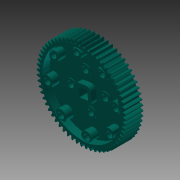
# Autodesk Inventor part: 276-2250
Saved by Autodesk Inventor 2013 (Build 170138000, 138)
## iProperties
Category: Motion
Company: Autodesk Inc.
Created: 2012-02-19
Part Number: 276-2250
Document SubType Name: Modeling
Designer: Autodesk Inc.
Density: 1.42 g/cm^3
Material: Acetal Resin, White
Catalog Web Link: http://www.vexrobotics.com/276-2250.html
Vendor: VEX
Mass: 21.4122 g
Surface Area: 169.555 cm^2
Volume: 15.079 cm^3
Author: Autodesk Inc.
Autodesk Inventor part; units mm, degrees
sketch "Sketch1" plane through (0, 0, 0) normal (0, 0, 1) x (1, 0, 0)
  arc A0 (28.1475, -11.53) -> (28.6057, -10.3412) centre (0, 0) ccw
  arc A1 (28.6057, -10.3412) -> (31.1315, -10.3412) centre (29.8686, -6.8477) ccw
  arc A2 (31.1315, -10.3412) -> (31.2381, -10.0146) centre (0, 0) ccw
  arc A3 (31.2381, -10.0146) -> (29.1986, -8.5246) centre (28.1575, -12.0904) ccw
  arc A4 (29.1986, -8.5246) -> (29.5299, -7.2944) centre (0, 0) ccw
  arc A5 (29.5299, -7.2944) -> (32.0419, -7.0304) centre (30.4207, -3.6881) ccw
  arc A6 (32.0419, -7.0304) -> (32.1137, -6.6945) centre (0, 0) ccw
  arc A7 (32.1137, -6.6945) -> (29.9297, -5.4258) centre (29.267, -9.081) ccw
  arc A8 (29.9297, -5.4258) -> (30.1306, -4.1677) centre (0, 0) ccw
  arc A9 (30.1306, -4.1677) -> (32.6012, -3.6426) centre (30.6396, -0.4881) ccw
  arc A10 (32.6012, -3.6426) -> (32.6376, -3.301) centre (0, 0) ccw
  arc A11 (32.6376, -3.301) -> (30.3329, -2.2676) centre (30.0559, -5.972) ccw
  arc A12 (30.3329, -2.2676) -> (30.4012, -0.9954) centre (0, 0) ccw
  arc A13 (30.4012, -0.9954) -> (32.8034, -0.2149) centre (30.5228, 2.7173) ccw
  arc A14 (32.8034, -0.2149) -> (32.8038, 0.1286) centre (0, 0) ccw
  arc A15 (32.8038, 0.1286) -> (30.4037, 0.9155) centre (30.5155, -2.7976) ccw
  arc A16 (30.4037, 0.9155) -> (30.3387, 2.1878) centre (0, 0) ccw
  arc A17 (30.3387, 2.1878) -> (32.6462, 3.2152) centre (30.0715, 5.8929) ccw
  arc A18 (32.6462, 3.2152) -> (32.6107, 3.5569) centre (0, 0) ccw
  arc A19 (32.6107, 3.5569) -> (30.1415, 4.0885) centre (30.6408, 0.4075) ccw
  arc A20 (30.1415, 4.0885) -> (29.9438, 5.3471) centre (0, 0) ccw
  arc A21 (29.9438, 5.3471) -> (32.1312, 6.61) centre (29.2908, 9.004) ccw
  arc A22 (32.1312, 6.61) -> (32.0603, 6.9461) centre (0, 0) ccw
  arc A23 (32.0603, 6.9461) -> (29.549, 7.2167) centre (30.4303, 3.6081) ccw
  arc A24 (29.549, 7.2167) -> (29.2209, 8.4478) centre (0, 0) ccw
  arc A25 (29.2209, 8.4478) -> (31.2643, 9.9324) centre (28.1892, 12.0164) ccw
  arc A26 (31.2643, 9.9324) -> (31.1586, 10.2593) centre (0, 0) ccw
  arc A27 (31.1586, 10.2593) -> (28.6328, 10.2659) centre (29.8865, 6.7692) ccw
  arc A28 (28.6328, 10.2659) -> (28.1778, 11.4559) centre (0, 0) ccw
  arc A29 (28.1778, 11.4559) -> (30.0548, 13.146) centre (26.7787, 14.8971) ccw
  arc A30 (30.0548, 13.146) -> (29.9155, 13.46) centre (0, 0) ccw
  arc A31 (29.9155, 13.46) -> (27.4028, 13.2026) centre (29.0152, 9.8561) ccw
  arc A32 (27.4028, 13.2026) -> (26.8259, 14.3386) centre (0, 0) ccw
  arc A33 (26.8259, 14.3386) -> (28.516, 16.2156) centre (25.0748, 17.6146) ccw
  arc A34 (28.516, 16.2156) -> (28.3446, 16.5133) centre (0, 0) ccw
  arc A35 (28.3446, 16.5133) -> (25.8727, 15.9947) centre (27.826, 12.835) ccw
  arc A36 (25.8727, 15.9947) -> (25.1802, 17.0641) centre (0, 0) ccw
  arc A37 (25.1802, 17.0641) -> (26.6648, 19.1075) centre (23.0962, 20.1392) ccw
  arc A38 (26.6648, 19.1075) -> (26.4633, 19.3857) centre (0, 0) ccw
  arc A39 (26.4633, 19.3857) -> (24.059, 18.6115) centre (26.3319, 15.6733) ccw
  arc A40 (24.059, 18.6115) -> (23.2586, 19.6026) centre (0, 0) ccw
  arc A41 (23.2586, 19.6026) -> (24.5215, 21.7901) centre (20.8646, 22.4431) ccw
  arc A42 (24.5215, 21.7901) -> (24.2919, 22.0457) centre (0, 0) ccw
  arc A43 (24.2919, 22.0457) -> (21.9818, 21.0244) centre (24.5494, 18.3399) ccw
  arc A44 (21.9818, 21.0244) -> (21.0821, 21.9264) centre (0, 0) ccw
  arc A45 (21.0821, 21.9264) -> (22.1094, 24.2339) centre (18.4044, 24.5011) ccw
  arc A46 (22.1094, 24.2339) -> (21.8545, 24.4641) centre (0, 0) ccw
  arc A47 (21.8545, 24.4641) -> (19.6637, 23.2069) centre (22.4979, 20.8055) ccw
  arc A48 (19.6637, 23.2069) -> (18.6747, 24.01) centre (0, 0) ccw
  arc A49 (18.6747, 24.01) -> (19.4552, 26.4122) centre (15.7425, 26.2906) ccw
  arc A50 (19.4552, 26.4122) -> (19.1776, 26.6145) centre (0, 0) ccw
  arc A51 (19.1776, 26.6145) -> (17.1302, 25.1352) centre (20.1998, 23.0432) ccw
  arc A52 (17.1302, 25.1352) -> (16.0627, 25.8305) centre (0, 0) ccw
  arc A53 (16.0627, 25.8305) -> (16.5878, 28.3011) centre (12.9081, 27.7921) ccw
  arc A54 (16.5878, 28.3011) -> (16.2905, 28.4733) centre (0, 0) ccw
  arc A55 (16.2905, 28.4733) -> (14.409, 26.7881) centre (17.6805, 25.0284) ccw
  arc A56 (14.409, 26.7881) -> (13.2746, 27.368) centre (0, 0) ccw
  arc A57 (13.2746, 27.368) -> (13.5387, 29.88) centre (9.9323, 28.9892) ccw
  arc A58 (13.5387, 29.88) -> (13.225, 30.0201) centre (0, 0) ccw
  arc A59 (13.225, 30.0201) -> (11.53, 28.1475) centre (14.9675, 26.7394) ccw
  arc A60 (11.53, 28.1475) -> (10.3412, 28.6057) centre (0, 0) ccw
  arc A61 (10.3412, 28.6057) -> (10.3412, 31.1315) centre (6.8477, 29.8686) ccw
  arc A62 (10.3412, 31.1315) -> (10.0146, 31.2381) centre (0, 0) ccw
  arc A63 (10.0146, 31.2381) -> (8.5246, 29.1986) centre (12.0904, 28.1575) ccw
  arc A64 (8.5246, 29.1986) -> (7.2944, 29.5299) centre (0, 0) ccw
  arc A65 (7.2944, 29.5299) -> (7.0304, 32.0419) centre (3.6881, 30.4207) ccw
  arc A66 (7.0304, 32.0419) -> (6.6945, 32.1137) centre (0, 0) ccw
  arc A67 (6.6945, 32.1137) -> (5.4258, 29.9297) centre (9.081, 29.267) ccw
  arc A68 (5.4258, 29.9297) -> (4.1677, 30.1306) centre (0, 0) ccw
  arc A69 (4.1677, 30.1306) -> (3.6426, 32.6012) centre (0.4881, 30.6396) ccw
  arc A70 (3.6426, 32.6012) -> (3.301, 32.6376) centre (0, 0) ccw
  arc A71 (3.301, 32.6376) -> (2.2676, 30.3329) centre (5.972, 30.0559) ccw
  arc A72 (2.2676, 30.3329) -> (0.9954, 30.4012) centre (0, 0) ccw
  arc A73 (0.9954, 30.4012) -> (0.2149, 32.8034) centre (-2.7173, 30.5228) ccw
  arc A74 (0.2149, 32.8034) -> (-0.1286, 32.8038) centre (0, 0) ccw
  arc A75 (-0.1286, 32.8038) -> (-0.9155, 30.4037) centre (2.7976, 30.5155) ccw
  arc A76 (-0.9155, 30.4037) -> (-2.1878, 30.3387) centre (0, 0) ccw
  arc A77 (-2.1878, 30.3387) -> (-3.2152, 32.6462) centre (-5.8929, 30.0715) ccw
  arc A78 (-3.2152, 32.6462) -> (-3.5569, 32.6107) centre (0, 0) ccw
  arc A79 (-3.5569, 32.6107) -> (-4.0885, 30.1415) centre (-0.4075, 30.6408) ccw
  arc A80 (-4.0885, 30.1415) -> (-5.3471, 29.9438) centre (0, 0) ccw
  arc A81 (-5.3471, 29.9438) -> (-6.61, 32.1312) centre (-9.004, 29.2908) ccw
  arc A82 (-6.61, 32.1312) -> (-6.9461, 32.0603) centre (0, 0) ccw
  arc A83 (-6.9461, 32.0603) -> (-7.2167, 29.549) centre (-3.6081, 30.4303) ccw
  arc A84 (-7.2167, 29.549) -> (-8.4478, 29.2209) centre (0, 0) ccw
  arc A85 (-8.4478, 29.2209) -> (-9.9324, 31.2643) centre (-12.0164, 28.1892) ccw
  arc A86 (-9.9324, 31.2643) -> (-10.2593, 31.1586) centre (0, 0) ccw
  arc A87 (-10.2593, 31.1586) -> (-10.2659, 28.6328) centre (-6.7692, 29.8865) ccw
  arc A88 (-10.2659, 28.6328) -> (-11.4559, 28.1778) centre (0, 0) ccw
  arc A89 (-11.4559, 28.1778) -> (-13.146, 30.0548) centre (-14.8971, 26.7787) ccw
  arc A90 (-13.146, 30.0548) -> (-13.46, 29.9155) centre (0, 0) ccw
  arc A91 (-13.46, 29.9155) -> (-13.2026, 27.4028) centre (-9.8561, 29.0152) ccw
  arc A92 (-13.2026, 27.4028) -> (-14.3386, 26.8259) centre (0, 0) ccw
  arc A93 (-14.3386, 26.8259) -> (-16.2156, 28.516) centre (-17.6146, 25.0748) ccw
  arc A94 (-16.2156, 28.516) -> (-16.5133, 28.3446) centre (0, 0) ccw
  arc A95 (-16.5133, 28.3446) -> (-15.9947, 25.8727) centre (-12.835, 27.826) ccw
  arc A96 (-15.9947, 25.8727) -> (-17.0641, 25.1802) centre (0, 0) ccw
  arc A97 (-17.0641, 25.1802) -> (-19.1075, 26.6648) centre (-20.1392, 23.0962) ccw
  arc A98 (-19.1075, 26.6648) -> (-19.3857, 26.4633) centre (0, 0) ccw
  arc A99 (-19.3857, 26.4633) -> (-18.6115, 24.059) centre (-15.6733, 26.3319) ccw
  arc A100 (-18.6115, 24.059) -> (-19.6026, 23.2586) centre (0, 0) ccw
  arc A101 (-19.6026, 23.2586) -> (-21.7901, 24.5215) centre (-22.4431, 20.8646) ccw
  arc A102 (-21.7901, 24.5215) -> (-22.0457, 24.2919) centre (0, 0) ccw
  arc A103 (-22.0457, 24.2919) -> (-21.0244, 21.9818) centre (-18.3399, 24.5494) ccw
  arc A104 (-21.0244, 21.9818) -> (-21.9264, 21.0821) centre (0, 0) ccw
  arc A105 (-21.9264, 21.0821) -> (-24.2339, 22.1094) centre (-24.5011, 18.4044) ccw
  arc A106 (-24.2339, 22.1094) -> (-24.4641, 21.8545) centre (0, 0) ccw
  arc A107 (-24.4641, 21.8545) -> (-23.2069, 19.6637) centre (-20.8055, 22.4979) ccw
  arc A108 (-23.2069, 19.6637) -> (-24.01, 18.6747) centre (0, 0) ccw
  arc A109 (-24.01, 18.6747) -> (-26.4122, 19.4552) centre (-26.2906, 15.7425) ccw
  arc A110 (-26.4122, 19.4552) -> (-26.6145, 19.1776) centre (0, 0) ccw
  arc A111 (-26.6145, 19.1776) -> (-25.1352, 17.1302) centre (-23.0432, 20.1998) ccw
  arc A112 (-25.1352, 17.1302) -> (-25.8305, 16.0627) centre (0, 0) ccw
  arc A113 (-25.8305, 16.0627) -> (-28.3011, 16.5878) centre (-27.7921, 12.9081) ccw
  arc A114 (-28.3011, 16.5878) -> (-28.4733, 16.2905) centre (0, 0) ccw
  arc A115 (-28.4733, 16.2905) -> (-26.7881, 14.409) centre (-25.0284, 17.6805) ccw
  arc A116 (-26.7881, 14.409) -> (-27.368, 13.2746) centre (0, 0) ccw
  arc A117 (-27.368, 13.2746) -> (-29.88, 13.5387) centre (-28.9892, 9.9323) ccw
  arc A118 (-29.88, 13.5387) -> (-30.0201, 13.225) centre (0, 0) ccw
  arc A119 (-30.0201, 13.225) -> (-28.1475, 11.53) centre (-26.7394, 14.9675) ccw
  arc A120 (-28.1475, 11.53) -> (-28.6057, 10.3412) centre (0, 0) ccw
  arc A121 (-28.6057, 10.3412) -> (-31.1315, 10.3412) centre (-29.8686, 6.8477) ccw
  arc A122 (-31.1315, 10.3412) -> (-31.2381, 10.0146) centre (0, 0) ccw
  arc A123 (-31.2381, 10.0146) -> (-29.1986, 8.5246) centre (-28.1575, 12.0904) ccw
  arc A124 (-29.1986, 8.5246) -> (-29.5299, 7.2944) centre (0, 0) ccw
  arc A125 (-29.5299, 7.2944) -> (-32.0419, 7.0304) centre (-30.4207, 3.6881) ccw
  arc A126 (-32.0419, 7.0304) -> (-32.1137, 6.6945) centre (0, 0) ccw
  arc A127 (-32.1137, 6.6945) -> (-29.9297, 5.4258) centre (-29.267, 9.081) ccw
  arc A128 (-29.9297, 5.4258) -> (-30.1306, 4.1677) centre (0, 0) ccw
  arc A129 (-30.1306, 4.1677) -> (-32.6012, 3.6426) centre (-30.6396, 0.4881) ccw
  arc A130 (-32.6012, 3.6426) -> (-32.6376, 3.301) centre (0, 0) ccw
  arc A131 (-32.6376, 3.301) -> (-30.3329, 2.2676) centre (-30.0559, 5.972) ccw
  arc A132 (-30.3329, 2.2676) -> (-30.4012, 0.9954) centre (0, 0) ccw
  arc A133 (-30.4012, 0.9954) -> (-32.8034, 0.2149) centre (-30.5228, -2.7173) ccw
  arc A134 (-32.8034, 0.2149) -> (-32.8038, -0.1286) centre (0, 0) ccw
  arc A135 (-32.8038, -0.1286) -> (-30.4037, -0.9155) centre (-30.5155, 2.7976) ccw
  arc A136 (-30.4037, -0.9155) -> (-30.3387, -2.1878) centre (0, 0) ccw
  arc A137 (-30.3387, -2.1878) -> (-32.6462, -3.2152) centre (-30.0715, -5.8929) ccw
  arc A138 (-32.6462, -3.2152) -> (-32.6107, -3.5569) centre (0, 0) ccw
  arc A139 (-32.6107, -3.5569) -> (-30.1415, -4.0885) centre (-30.6408, -0.4075) ccw
  arc A140 (-30.1415, -4.0885) -> (-29.9438, -5.3471) centre (0, 0) ccw
  arc A141 (-29.9438, -5.3471) -> (-32.1312, -6.61) centre (-29.2908, -9.004) ccw
  arc A142 (-32.1312, -6.61) -> (-32.0603, -6.9461) centre (0, 0) ccw
  arc A143 (-32.0603, -6.9461) -> (-29.549, -7.2167) centre (-30.4303, -3.6081) ccw
  arc A144 (-29.549, -7.2167) -> (-29.2209, -8.4478) centre (0, 0) ccw
  arc A145 (-29.2209, -8.4478) -> (-31.2643, -9.9324) centre (-28.1892, -12.0164) ccw
  arc A146 (-31.2643, -9.9324) -> (-31.1586, -10.2593) centre (0, 0) ccw
  arc A147 (-31.1586, -10.2593) -> (-28.6328, -10.2659) centre (-29.8865, -6.7692) ccw
  arc A148 (-28.6328, -10.2659) -> (-28.1778, -11.4559) centre (0, 0) ccw
  arc A149 (-28.1778, -11.4559) -> (-30.0548, -13.146) centre (-26.7787, -14.8971) ccw
  arc A150 (-30.0548, -13.146) -> (-29.9155, -13.46) centre (0, 0) ccw
  arc A151 (-29.9155, -13.46) -> (-27.4028, -13.2026) centre (-29.0152, -9.8561) ccw
  arc A152 (-27.4028, -13.2026) -> (-26.8259, -14.3386) centre (0, 0) ccw
  arc A153 (-26.8259, -14.3386) -> (-28.516, -16.2156) centre (-25.0748, -17.6146) ccw
  arc A154 (-28.516, -16.2156) -> (-28.3446, -16.5133) centre (0, 0) ccw
  arc A155 (-28.3446, -16.5133) -> (-25.8727, -15.9947) centre (-27.826, -12.835) ccw
  arc A156 (-25.8727, -15.9947) -> (-25.1802, -17.0641) centre (0, 0) ccw
  arc A157 (-25.1802, -17.0641) -> (-26.6648, -19.1075) centre (-23.0962, -20.1392) ccw
  arc A158 (-26.6648, -19.1075) -> (-26.4633, -19.3857) centre (0, 0) ccw
  arc A159 (-26.4633, -19.3857) -> (-24.059, -18.6115) centre (-26.3319, -15.6733) ccw
  arc A160 (-24.059, -18.6115) -> (-23.2586, -19.6026) centre (0, 0) ccw
  arc A161 (-23.2586, -19.6026) -> (-24.5215, -21.7901) centre (-20.8646, -22.4431) ccw
  arc A162 (-24.5215, -21.7901) -> (-24.2919, -22.0457) centre (0, 0) ccw
  arc A163 (-24.2919, -22.0457) -> (-21.9818, -21.0244) centre (-24.5494, -18.3399) ccw
  arc A164 (-21.9818, -21.0244) -> (-21.0821, -21.9264) centre (0, 0) ccw
  arc A165 (-21.0821, -21.9264) -> (-22.1094, -24.2339) centre (-18.4044, -24.5011) ccw
  arc A166 (-22.1094, -24.2339) -> (-21.8545, -24.4641) centre (0, 0) ccw
  arc A167 (-21.8545, -24.4641) -> (-19.6637, -23.2069) centre (-22.4979, -20.8055) ccw
  arc A168 (-19.6637, -23.2069) -> (-18.6747, -24.01) centre (0, 0) ccw
  arc A169 (-18.6747, -24.01) -> (-19.4552, -26.4122) centre (-15.7425, -26.2906) ccw
  arc A170 (-19.4552, -26.4122) -> (-19.1776, -26.6145) centre (0, 0) ccw
  arc A171 (-19.1776, -26.6145) -> (-17.1302, -25.1352) centre (-20.1998, -23.0432) ccw
  arc A172 (-17.1302, -25.1352) -> (-16.0627, -25.8305) centre (0, 0) ccw
  arc A173 (-16.0627, -25.8305) -> (-16.5878, -28.3011) centre (-12.9081, -27.7921) ccw
  arc A174 (-16.5878, -28.3011) -> (-16.2905, -28.4733) centre (0, 0) ccw
  arc A175 (-16.2905, -28.4733) -> (-14.409, -26.7881) centre (-17.6805, -25.0284) ccw
  arc A176 (-14.409, -26.7881) -> (-13.2746, -27.368) centre (0, 0) ccw
  arc A177 (-13.2746, -27.368) -> (-13.5387, -29.88) centre (-9.9323, -28.9892) ccw
  arc A178 (-13.5387, -29.88) -> (-13.225, -30.0201) centre (0, 0) ccw
  arc A179 (-13.225, -30.0201) -> (-11.53, -28.1475) centre (-14.9675, -26.7394) ccw
  arc A180 (-11.53, -28.1475) -> (-10.3412, -28.6057) centre (0, 0) ccw
  arc A181 (-10.3412, -28.6057) -> (-10.3412, -31.1315) centre (-6.8477, -29.8686) ccw
  arc A182 (-10.3412, -31.1315) -> (-10.0146, -31.2381) centre (0, 0) ccw
  arc A183 (-10.0146, -31.2381) -> (-8.5246, -29.1986) centre (-12.0904, -28.1575) ccw
  arc A184 (-8.5246, -29.1986) -> (-7.2944, -29.5299) centre (0, 0) ccw
  arc A185 (-7.2944, -29.5299) -> (-7.0304, -32.0419) centre (-3.6881, -30.4207) ccw
  arc A186 (-7.0304, -32.0419) -> (-6.6945, -32.1137) centre (0, 0) ccw
  arc A187 (-6.6945, -32.1137) -> (-5.4258, -29.9297) centre (-9.081, -29.267) ccw
  arc A188 (-5.4258, -29.9297) -> (-4.1677, -30.1306) centre (0, 0) ccw
  arc A189 (-4.1677, -30.1306) -> (-3.6426, -32.6012) centre (-0.4881, -30.6396) ccw
  arc A190 (-3.6426, -32.6012) -> (-3.301, -32.6376) centre (0, 0) ccw
  arc A191 (-3.301, -32.6376) -> (-2.2676, -30.3329) centre (-5.972, -30.0559) ccw
  arc A192 (-2.2676, -30.3329) -> (-0.9954, -30.4012) centre (0, 0) ccw
  arc A193 (-0.9954, -30.4012) -> (-0.2149, -32.8034) centre (2.7173, -30.5228) ccw
  arc A194 (-0.2149, -32.8034) -> (0.1286, -32.8038) centre (0, 0) ccw
  arc A195 (0.1286, -32.8038) -> (0.9155, -30.4037) centre (-2.7976, -30.5155) ccw
  arc A196 (0.9155, -30.4037) -> (2.1878, -30.3387) centre (0, 0) ccw
  arc A197 (2.1878, -30.3387) -> (3.2152, -32.6462) centre (5.8929, -30.0715) ccw
  arc A198 (3.2152, -32.6462) -> (3.5569, -32.6107) centre (0, 0) ccw
  arc A199 (3.5569, -32.6107) -> (4.0885, -30.1415) centre (0.4075, -30.6408) ccw
  arc A200 (4.0885, -30.1415) -> (5.3471, -29.9438) centre (0, 0) ccw
  arc A201 (5.3471, -29.9438) -> (6.61, -32.1312) centre (9.004, -29.2908) ccw
  arc A202 (6.61, -32.1312) -> (6.9461, -32.0603) centre (0, 0) ccw
  arc A203 (6.9461, -32.0603) -> (7.2167, -29.549) centre (3.6081, -30.4303) ccw
  arc A204 (7.2167, -29.549) -> (8.4478, -29.2209) centre (0, 0) ccw
  arc A205 (8.4478, -29.2209) -> (9.9324, -31.2643) centre (12.0164, -28.1892) ccw
  arc A206 (9.9324, -31.2643) -> (10.2593, -31.1586) centre (0, 0) ccw
  arc A207 (10.2593, -31.1586) -> (10.2659, -28.6328) centre (6.7692, -29.8865) ccw
  arc A208 (10.2659, -28.6328) -> (11.4559, -28.1778) centre (0, 0) ccw
  arc A209 (11.4559, -28.1778) -> (13.146, -30.0548) centre (14.8971, -26.7787) ccw
  arc A210 (13.146, -30.0548) -> (13.46, -29.9155) centre (0, 0) ccw
  arc A211 (13.46, -29.9155) -> (13.2026, -27.4028) centre (9.8561, -29.0152) ccw
  arc A212 (13.2026, -27.4028) -> (14.3386, -26.8259) centre (0, 0) ccw
  arc A213 (14.3386, -26.8259) -> (16.2156, -28.516) centre (17.6146, -25.0748) ccw
  arc A214 (16.2156, -28.516) -> (16.5133, -28.3446) centre (0, 0) ccw
  arc A215 (16.5133, -28.3446) -> (15.9947, -25.8727) centre (12.835, -27.826) ccw
  arc A216 (15.9947, -25.8727) -> (17.0641, -25.1802) centre (0, 0) ccw
  arc A217 (17.0641, -25.1802) -> (19.1075, -26.6648) centre (20.1392, -23.0962) ccw
  arc A218 (19.1075, -26.6648) -> (19.3857, -26.4633) centre (0, 0) ccw
  arc A219 (19.3857, -26.4633) -> (18.6115, -24.059) centre (15.6733, -26.3319) ccw
  arc A220 (18.6115, -24.059) -> (19.6026, -23.2586) centre (0, 0) ccw
  arc A221 (19.6026, -23.2586) -> (21.7901, -24.5215) centre (22.4431, -20.8646) ccw
  arc A222 (21.7901, -24.5215) -> (22.0457, -24.2919) centre (0, 0) ccw
  arc A223 (22.0457, -24.2919) -> (21.0244, -21.9818) centre (18.3399, -24.5494) ccw
  arc A224 (21.0244, -21.9818) -> (21.9264, -21.0821) centre (0, 0) ccw
  arc A225 (21.9264, -21.0821) -> (24.2339, -22.1094) centre (24.5011, -18.4044) ccw
  arc A226 (24.2339, -22.1094) -> (24.4641, -21.8545) centre (0, 0) ccw
  arc A227 (24.4641, -21.8545) -> (23.2069, -19.6637) centre (20.8055, -22.4979) ccw
  arc A228 (23.2069, -19.6637) -> (24.01, -18.6747) centre (0, 0) ccw
  arc A229 (24.01, -18.6747) -> (26.4122, -19.4552) centre (26.2906, -15.7425) ccw
  arc A230 (26.4122, -19.4552) -> (26.6145, -19.1776) centre (0, 0) ccw
  arc A231 (26.6145, -19.1776) -> (25.1352, -17.1302) centre (23.0432, -20.1998) ccw
  arc A232 (25.1352, -17.1302) -> (25.8305, -16.0627) centre (0, 0) ccw
  arc A233 (25.8305, -16.0627) -> (28.3011, -16.5878) centre (27.7921, -12.9081) ccw
  arc A234 (28.3011, -16.5878) -> (28.4733, -16.2905) centre (0, 0) ccw
  arc A235 (28.4733, -16.2905) -> (26.7881, -14.409) centre (25.0284, -17.6805) ccw
  arc A236 (26.7881, -14.409) -> (27.368, -13.2746) centre (0, 0) ccw
  arc A237 (27.368, -13.2746) -> (29.88, -13.5387) centre (28.9892, -9.9323) ccw
  arc A238 (29.88, -13.5387) -> (30.0201, -13.225) centre (0, 0) ccw
  arc A239 (30.0201, -13.225) -> (28.1475, -11.53) centre (26.7394, -14.9675) ccw
  arc A240 (-19.6657, 20.5138) -> (-25.5542, 12.4313) centre (-7.1656, 5.2205) ccw
  arc A241 (-9.2793, 26.8598) -> (-19.6657, 20.5138) centre (0, 0) ccw
  arc A242 (0.5997, 28.4112) -> (-9.2793, 26.8598) centre (-1.3754, 8.7583) ccw
  arc A243 (12.4313, 25.5542) -> (0.5997, 28.4112) centre (0, 0) ccw
  arc A244 (20.5138, 19.6657) -> (12.4313, 25.5542) centre (5.2205, 7.1656) ccw
  arc A245 (26.8598, 9.2793) -> (20.5138, 19.6657) centre (0, 0) ccw
  arc A246 (28.4112, -0.5997) -> (26.8598, 9.2793) centre (8.7583, 1.3754) ccw
  arc A247 (25.5542, -12.4313) -> (28.4112, -0.5997) centre (0, 0) ccw
  arc A248 (19.6657, -20.5138) -> (25.5542, -12.4313) centre (7.1656, -5.2205) ccw
  arc A249 (9.2793, -26.8598) -> (19.6657, -20.5138) centre (0, 0) ccw
  arc A250 (-0.5997, -28.4112) -> (9.2793, -26.8598) centre (1.3754, -8.7583) ccw
  arc A251 (-12.4313, -25.5542) -> (-0.5997, -28.4112) centre (0, 0) ccw
  arc A252 (-20.5138, -19.6657) -> (-12.4313, -25.5542) centre (-5.2205, -7.1656) ccw
  arc A253 (-26.8598, -9.2793) -> (-20.5138, -19.6657) centre (0, 0) ccw
  arc A254 (-28.4112, 0.5997) -> (-26.8598, -9.2793) centre (-8.7583, -1.3754) ccw
  arc A255 (-25.5542, 12.4313) -> (-28.4112, 0.5997) centre (0, 0) ccw
  arc A256 (-11.7238, -22.8848) -> (-18.1897, -18.174) centre (-14.9567, -20.5294) ccw
  arc A257 (-18.1897, -18.174) -> (-11.7238, -22.8848) centre (-13.9277, -19.1169) ccw
  arc A258 (-18.174, 18.1897) -> (-22.8848, 11.7238) centre (-19.1169, 13.9277) ccw
  arc A259 (-22.8848, 11.7238) -> (-18.174, 18.1897) centre (-20.5294, 14.9567) ccw
  arc A260 (-7.892, 24.4719) -> (0.0111, 25.713) centre (-3.9404, 25.0925) ccw
  arc A261 (0.0111, 25.713) -> (-7.892, 24.4719) centre (-3.6693, 23.366) ccw
  arc A262 (18.1897, 18.174) -> (11.7238, 22.8848) centre (13.9277, 19.1169) ccw
  arc A263 (11.7238, 22.8848) -> (18.1897, 18.174) centre (14.9567, 20.5294) ccw
  arc A264 (22.8848, -11.7238) -> (18.174, -18.1897) centre (20.5294, -14.9567) ccw
  arc A265 (18.174, -18.1897) -> (22.8848, -11.7238) centre (19.1169, -13.9277) ccw
  circle A266 centre (-14.9567, -20.5294) radius 2.2225
  circle A267 centre (-25.0925, -3.9404) radius 2.2225
  circle A268 centre (-20.5294, 14.9567) radius 2.2225
  circle A269 centre (-3.9404, 25.0925) radius 2.2225
  circle A270 centre (14.9567, 20.5294) radius 2.2225
  circle A271 centre (25.0925, 3.9404) radius 2.2225
  circle A272 centre (20.5294, -14.9567) radius 2.2225
  circle A273 centre (3.9404, -25.0925) radius 2.2225
  arc A274 (28.1475, -11.53) -> (28.6057, -10.3412) centre (0, 0) ccw
  arc A275 (30.0201, -13.225) -> (28.1475, -11.53) centre (26.7394, -14.9675) ccw
  arc A276 (29.88, -13.5387) -> (30.0201, -13.225) centre (0, 0) ccw
  arc A277 (27.368, -13.2746) -> (29.88, -13.5387) centre (28.9892, -9.9323) ccw
  arc A278 (26.7881, -14.409) -> (27.368, -13.2746) centre (0, 0) ccw
  arc A279 (28.4733, -16.2905) -> (26.7881, -14.409) centre (25.0284, -17.6805) ccw
  arc A280 (28.3011, -16.5878) -> (28.4733, -16.2905) centre (0, 0) ccw
  arc A281 (25.8305, -16.0627) -> (28.3011, -16.5878) centre (27.7921, -12.9081) ccw
  arc A282 (25.1352, -17.1302) -> (25.8305, -16.0627) centre (0, 0) ccw
  arc A283 (26.6145, -19.1776) -> (25.1352, -17.1302) centre (23.0432, -20.1998) ccw
  arc A284 (26.4122, -19.4552) -> (26.6145, -19.1776) centre (0, 0) ccw
  arc A285 (24.01, -18.6747) -> (26.4122, -19.4552) centre (26.2906, -15.7425) ccw
  arc A286 (23.2069, -19.6637) -> (24.01, -18.6747) centre (0, 0) ccw
  arc A287 (24.4641, -21.8545) -> (23.2069, -19.6637) centre (20.8055, -22.4979) ccw
  arc A288 (24.2339, -22.1094) -> (24.4641, -21.8545) centre (0, 0) ccw
  arc A289 (21.9264, -21.0821) -> (24.2339, -22.1094) centre (24.5011, -18.4044) ccw
  arc A290 (21.0244, -21.9818) -> (21.9264, -21.0821) centre (0, 0) ccw
  arc A291 (22.0457, -24.2919) -> (21.0244, -21.9818) centre (18.3399, -24.5494) ccw
  arc A292 (21.7901, -24.5215) -> (22.0457, -24.2919) centre (0, 0) ccw
  arc A293 (19.6026, -23.2586) -> (21.7901, -24.5215) centre (22.4431, -20.8646) ccw
  arc A294 (18.6115, -24.059) -> (19.6026, -23.2586) centre (0, 0) ccw
  arc A295 (19.3857, -26.4633) -> (18.6115, -24.059) centre (15.6733, -26.3319) ccw
  arc A296 (19.1075, -26.6648) -> (19.3857, -26.4633) centre (0, 0) ccw
  arc A297 (17.0641, -25.1802) -> (19.1075, -26.6648) centre (20.1392, -23.0962) ccw
  arc A298 (15.9947, -25.8727) -> (17.0641, -25.1802) centre (0, 0) ccw
  arc A299 (16.5133, -28.3446) -> (15.9947, -25.8727) centre (12.835, -27.826) ccw
  arc A300 (16.2156, -28.516) -> (16.5133, -28.3446) centre (0, 0) ccw
  arc A301 (14.3386, -26.8259) -> (16.2156, -28.516) centre (17.6146, -25.0748) ccw
  arc A302 (13.2026, -27.4028) -> (14.3386, -26.8259) centre (0, 0) ccw
  arc A303 (13.46, -29.9155) -> (13.2026, -27.4028) centre (9.8561, -29.0152) ccw
  arc A304 (13.146, -30.0548) -> (13.46, -29.9155) centre (0, 0) ccw
  arc A305 (11.4559, -28.1778) -> (13.146, -30.0548) centre (14.8971, -26.7787) ccw
  arc A306 (10.2659, -28.6328) -> (11.4559, -28.1778) centre (0, 0) ccw
  arc A307 (10.2593, -31.1586) -> (10.2659, -28.6328) centre (6.7692, -29.8865) ccw
  arc A308 (9.9324, -31.2643) -> (10.2593, -31.1586) centre (0, 0) ccw
  arc A309 (8.4478, -29.2209) -> (9.9324, -31.2643) centre (12.0164, -28.1892) ccw
  arc A310 (7.2167, -29.549) -> (8.4478, -29.2209) centre (0, 0) ccw
  arc A311 (6.9461, -32.0603) -> (7.2167, -29.549) centre (3.6081, -30.4303) ccw
  arc A312 (6.61, -32.1312) -> (6.9461, -32.0603) centre (0, 0) ccw
  arc A313 (5.3471, -29.9438) -> (6.61, -32.1312) centre (9.004, -29.2908) ccw
  arc A314 (4.0885, -30.1415) -> (5.3471, -29.9438) centre (0, 0) ccw
  arc A315 (3.5569, -32.6107) -> (4.0885, -30.1415) centre (0.4075, -30.6408) ccw
  arc A316 (3.2152, -32.6462) -> (3.5569, -32.6107) centre (0, 0) ccw
  arc A317 (2.1878, -30.3387) -> (3.2152, -32.6462) centre (5.8929, -30.0715) ccw
  arc A318 (0.9155, -30.4037) -> (2.1878, -30.3387) centre (0, 0) ccw
  arc A319 (0.1286, -32.8038) -> (0.9155, -30.4037) centre (-2.7976, -30.5155) ccw
  arc A320 (-0.2149, -32.8034) -> (0.1286, -32.8038) centre (0, 0) ccw
  arc A321 (-0.9954, -30.4012) -> (-0.2149, -32.8034) centre (2.7173, -30.5228) ccw
  arc A322 (-2.2676, -30.3329) -> (-0.9954, -30.4012) centre (0, 0) ccw
  arc A323 (-3.301, -32.6376) -> (-2.2676, -30.3329) centre (-5.972, -30.0559) ccw
  arc A324 (-3.6426, -32.6012) -> (-3.301, -32.6376) centre (0, 0) ccw
  arc A325 (-4.1677, -30.1306) -> (-3.6426, -32.6012) centre (-0.4881, -30.6396) ccw
  arc A326 (-5.4258, -29.9297) -> (-4.1677, -30.1306) centre (0, 0) ccw
  arc A327 (-6.6945, -32.1137) -> (-5.4258, -29.9297) centre (-9.081, -29.267) ccw
  arc A328 (-7.0304, -32.0419) -> (-6.6945, -32.1137) centre (0, 0) ccw
  arc A329 (-7.2944, -29.5299) -> (-7.0304, -32.0419) centre (-3.6881, -30.4207) ccw
  arc A330 (-8.5246, -29.1986) -> (-7.2944, -29.5299) centre (0, 0) ccw
  arc A331 (-10.0146, -31.2381) -> (-8.5246, -29.1986) centre (-12.0904, -28.1575) ccw
  arc A332 (-10.3412, -31.1315) -> (-10.0146, -31.2381) centre (0, 0) ccw
  arc A333 (-10.3412, -28.6057) -> (-10.3412, -31.1315) centre (-6.8477, -29.8686) ccw
  arc A334 (-11.53, -28.1475) -> (-10.3412, -28.6057) centre (0, 0) ccw
  arc A335 (-13.225, -30.0201) -> (-11.53, -28.1475) centre (-14.9675, -26.7394) ccw
  arc A336 (-13.5387, -29.88) -> (-13.225, -30.0201) centre (0, 0) ccw
  arc A337 (-13.2746, -27.368) -> (-13.5387, -29.88) centre (-9.9323, -28.9892) ccw
  arc A338 (-14.409, -26.7881) -> (-13.2746, -27.368) centre (0, 0) ccw
  arc A339 (-16.2905, -28.4733) -> (-14.409, -26.7881) centre (-17.6805, -25.0284) ccw
  arc A340 (-16.5878, -28.3011) -> (-16.2905, -28.4733) centre (0, 0) ccw
  arc A341 (-16.0627, -25.8305) -> (-16.5878, -28.3011) centre (-12.9081, -27.7921) ccw
  arc A342 (-17.1302, -25.1352) -> (-16.0627, -25.8305) centre (0, 0) ccw
  arc A343 (-19.1776, -26.6145) -> (-17.1302, -25.1352) centre (-20.1998, -23.0432) ccw
  arc A344 (-19.4552, -26.4122) -> (-19.1776, -26.6145) centre (0, 0) ccw
  arc A345 (-18.6747, -24.01) -> (-19.4552, -26.4122) centre (-15.7425, -26.2906) ccw
  arc A346 (-19.6637, -23.2069) -> (-18.6747, -24.01) centre (0, 0) ccw
  arc A347 (-21.8545, -24.4641) -> (-19.6637, -23.2069) centre (-22.4979, -20.8055) ccw
  arc A348 (-22.1094, -24.2339) -> (-21.8545, -24.4641) centre (0, 0) ccw
  arc A349 (-21.0821, -21.9264) -> (-22.1094, -24.2339) centre (-18.4044, -24.5011) ccw
  arc A350 (-21.9818, -21.0244) -> (-21.0821, -21.9264) centre (0, 0) ccw
  arc A351 (-24.2919, -22.0457) -> (-21.9818, -21.0244) centre (-24.5494, -18.3399) ccw
  arc A352 (-24.5215, -21.7901) -> (-24.2919, -22.0457) centre (0, 0) ccw
  arc A353 (-23.2586, -19.6026) -> (-24.5215, -21.7901) centre (-20.8646, -22.4431) ccw
  arc A354 (-24.059, -18.6115) -> (-23.2586, -19.6026) centre (0, 0) ccw
  arc A355 (-26.4633, -19.3857) -> (-24.059, -18.6115) centre (-26.3319, -15.6733) ccw
  arc A356 (-26.6648, -19.1075) -> (-26.4633, -19.3857) centre (0, 0) ccw
  arc A357 (-25.1802, -17.0641) -> (-26.6648, -19.1075) centre (-23.0962, -20.1392) ccw
  arc A358 (-25.8727, -15.9947) -> (-25.1802, -17.0641) centre (0, 0) ccw
  arc A359 (-28.3446, -16.5133) -> (-25.8727, -15.9947) centre (-27.826, -12.835) ccw
  arc A360 (-28.516, -16.2156) -> (-28.3446, -16.5133) centre (0, 0) ccw
  arc A361 (-26.8259, -14.3386) -> (-28.516, -16.2156) centre (-25.0748, -17.6146) ccw
  arc A362 (-27.4028, -13.2026) -> (-26.8259, -14.3386) centre (0, 0) ccw
  arc A363 (-29.9155, -13.46) -> (-27.4028, -13.2026) centre (-29.0152, -9.8561) ccw
  arc A364 (-30.0548, -13.146) -> (-29.9155, -13.46) centre (0, 0) ccw
  arc A365 (-28.1778, -11.4559) -> (-30.0548, -13.146) centre (-26.7787, -14.8971) ccw
  arc A366 (-28.6328, -10.2659) -> (-28.1778, -11.4559) centre (0, 0) ccw
  arc A367 (-31.1586, -10.2593) -> (-28.6328, -10.2659) centre (-29.8865, -6.7692) ccw
  arc A368 (-31.2643, -9.9324) -> (-31.1586, -10.2593) centre (0, 0) ccw
  arc A369 (-29.2209, -8.4478) -> (-31.2643, -9.9324) centre (-28.1892, -12.0164) ccw
  arc A370 (-29.549, -7.2167) -> (-29.2209, -8.4478) centre (0, 0) ccw
  arc A371 (-32.0603, -6.9461) -> (-29.549, -7.2167) centre (-30.4303, -3.6081) ccw
  arc A372 (-32.1312, -6.61) -> (-32.0603, -6.9461) centre (0, 0) ccw
  arc A373 (-29.9438, -5.3471) -> (-32.1312, -6.61) centre (-29.2908, -9.004) ccw
  arc A374 (-30.1415, -4.0885) -> (-29.9438, -5.3471) centre (0, 0) ccw
  arc A375 (-32.6107, -3.5569) -> (-30.1415, -4.0885) centre (-30.6408, -0.4075) ccw
  arc A376 (-32.6462, -3.2152) -> (-32.6107, -3.5569) centre (0, 0) ccw
  arc A377 (-30.3387, -2.1878) -> (-32.6462, -3.2152) centre (-30.0715, -5.8929) ccw
  arc A378 (-30.4037, -0.9155) -> (-30.3387, -2.1878) centre (0, 0) ccw
  arc A379 (-32.8038, -0.1286) -> (-30.4037, -0.9155) centre (-30.5155, 2.7976) ccw
  arc A380 (-32.8034, 0.2149) -> (-32.8038, -0.1286) centre (0, 0) ccw
  arc A381 (-30.4012, 0.9954) -> (-32.8034, 0.2149) centre (-30.5228, -2.7173) ccw
  arc A382 (-30.3329, 2.2676) -> (-30.4012, 0.9954) centre (0, 0) ccw
  arc A383 (-32.6376, 3.301) -> (-30.3329, 2.2676) centre (-30.0559, 5.972) ccw
  arc A384 (-32.6012, 3.6426) -> (-32.6376, 3.301) centre (0, 0) ccw
  arc A385 (-30.1306, 4.1677) -> (-32.6012, 3.6426) centre (-30.6396, 0.4881) ccw
  arc A386 (-29.9297, 5.4258) -> (-30.1306, 4.1677) centre (0, 0) ccw
  arc A387 (-32.1137, 6.6945) -> (-29.9297, 5.4258) centre (-29.267, 9.081) ccw
  arc A388 (-32.0419, 7.0304) -> (-32.1137, 6.6945) centre (0, 0) ccw
  arc A389 (-29.5299, 7.2944) -> (-32.0419, 7.0304) centre (-30.4207, 3.6881) ccw
  arc A390 (-29.1986, 8.5246) -> (-29.5299, 7.2944) centre (0, 0) ccw
  arc A391 (-31.2381, 10.0146) -> (-29.1986, 8.5246) centre (-28.1575, 12.0904) ccw
  arc A392 (-31.1315, 10.3412) -> (-31.2381, 10.0146) centre (0, 0) ccw
  arc A393 (-28.6057, 10.3412) -> (-31.1315, 10.3412) centre (-29.8686, 6.8477) ccw
  arc A394 (-28.1475, 11.53) -> (-28.6057, 10.3412) centre (0, 0) ccw
  arc A395 (-30.0201, 13.225) -> (-28.1475, 11.53) centre (-26.7394, 14.9675) ccw
  arc A396 (-29.88, 13.5387) -> (-30.0201, 13.225) centre (0, 0) ccw
  arc A397 (-27.368, 13.2746) -> (-29.88, 13.5387) centre (-28.9892, 9.9323) ccw
  arc A398 (-26.7881, 14.409) -> (-27.368, 13.2746) centre (0, 0) ccw
  arc A399 (-28.4733, 16.2905) -> (-26.7881, 14.409) centre (-25.0284, 17.6805) ccw
  arc A400 (-28.3011, 16.5878) -> (-28.4733, 16.2905) centre (0, 0) ccw
  arc A401 (-25.8305, 16.0627) -> (-28.3011, 16.5878) centre (-27.7921, 12.9081) ccw
  arc A402 (-25.1352, 17.1302) -> (-25.8305, 16.0627) centre (0, 0) ccw
  arc A403 (-26.6145, 19.1776) -> (-25.1352, 17.1302) centre (-23.0432, 20.1998) ccw
  arc A404 (-26.4122, 19.4552) -> (-26.6145, 19.1776) centre (0, 0) ccw
  arc A405 (-24.01, 18.6747) -> (-26.4122, 19.4552) centre (-26.2906, 15.7425) ccw
  arc A406 (-23.2069, 19.6637) -> (-24.01, 18.6747) centre (0, 0) ccw
  arc A407 (-24.4641, 21.8545) -> (-23.2069, 19.6637) centre (-20.8055, 22.4979) ccw
  arc A408 (-24.2339, 22.1094) -> (-24.4641, 21.8545) centre (0, 0) ccw
  arc A409 (-21.9264, 21.0821) -> (-24.2339, 22.1094) centre (-24.5011, 18.4044) ccw
  arc A410 (-21.0244, 21.9818) -> (-21.9264, 21.0821) centre (0, 0) ccw
  arc A411 (-22.0457, 24.2919) -> (-21.0244, 21.9818) centre (-18.3399, 24.5494) ccw
  arc A412 (-21.7901, 24.5215) -> (-22.0457, 24.2919) centre (0, 0) ccw
  arc A413 (-19.6026, 23.2586) -> (-21.7901, 24.5215) centre (-22.4431, 20.8646) ccw
  arc A414 (-18.6115, 24.059) -> (-19.6026, 23.2586) centre (0, 0) ccw
  arc A415 (-19.3857, 26.4633) -> (-18.6115, 24.059) centre (-15.6733, 26.3319) ccw
  arc A416 (-19.1075, 26.6648) -> (-19.3857, 26.4633) centre (0, 0) ccw
  arc A417 (-17.0641, 25.1802) -> (-19.1075, 26.6648) centre (-20.1392, 23.0962) ccw
  arc A418 (-15.9947, 25.8727) -> (-17.0641, 25.1802) centre (0, 0) ccw
  arc A419 (-16.5133, 28.3446) -> (-15.9947, 25.8727) centre (-12.835, 27.826) ccw
  arc A420 (-16.2156, 28.516) -> (-16.5133, 28.3446) centre (0, 0) ccw
  arc A421 (-14.3386, 26.8259) -> (-16.2156, 28.516) centre (-17.6146, 25.0748) ccw
  arc A422 (-13.2026, 27.4028) -> (-14.3386, 26.8259) centre (0, 0) ccw
  arc A423 (-13.46, 29.9155) -> (-13.2026, 27.4028) centre (-9.8561, 29.0152) ccw
  arc A424 (-13.146, 30.0548) -> (-13.46, 29.9155) centre (0, 0) ccw
  arc A425 (-11.4559, 28.1778) -> (-13.146, 30.0548) centre (-14.8971, 26.7787) ccw
  arc A426 (-10.2659, 28.6328) -> (-11.4559, 28.1778) centre (0, 0) ccw
  arc A427 (-10.2593, 31.1586) -> (-10.2659, 28.6328) centre (-6.7692, 29.8865) ccw
  arc A428 (-9.9324, 31.2643) -> (-10.2593, 31.1586) centre (0, 0) ccw
  arc A429 (-8.4478, 29.2209) -> (-9.9324, 31.2643) centre (-12.0164, 28.1892) ccw
  arc A430 (-7.2167, 29.549) -> (-8.4478, 29.2209) centre (0, 0) ccw
  arc A431 (-6.9461, 32.0603) -> (-7.2167, 29.549) centre (-3.6081, 30.4303) ccw
  arc A432 (-6.61, 32.1312) -> (-6.9461, 32.0603) centre (0, 0) ccw
  arc A433 (-5.3471, 29.9438) -> (-6.61, 32.1312) centre (-9.004, 29.2908) ccw
  arc A434 (-4.0885, 30.1415) -> (-5.3471, 29.9438) centre (0, 0) ccw
  arc A435 (-3.5569, 32.6107) -> (-4.0885, 30.1415) centre (-0.4075, 30.6408) ccw
  arc A436 (-3.2152, 32.6462) -> (-3.5569, 32.6107) centre (0, 0) ccw
  arc A437 (-2.1878, 30.3387) -> (-3.2152, 32.6462) centre (-5.8929, 30.0715) ccw
  arc A438 (-0.9155, 30.4037) -> (-2.1878, 30.3387) centre (0, 0) ccw
  arc A439 (-0.1286, 32.8038) -> (-0.9155, 30.4037) centre (2.7976, 30.5155) ccw
  arc A440 (0.2149, 32.8034) -> (-0.1286, 32.8038) centre (0, 0) ccw
  arc A441 (0.9954, 30.4012) -> (0.2149, 32.8034) centre (-2.7173, 30.5228) ccw
  arc A442 (2.2676, 30.3329) -> (0.9954, 30.4012) centre (0, 0) ccw
  arc A443 (3.301, 32.6376) -> (2.2676, 30.3329) centre (5.972, 30.0559) ccw
  arc A444 (3.6426, 32.6012) -> (3.301, 32.6376) centre (0, 0) ccw
  arc A445 (4.1677, 30.1306) -> (3.6426, 32.6012) centre (0.4881, 30.6396) ccw
  arc A446 (5.4258, 29.9297) -> (4.1677, 30.1306) centre (0, 0) ccw
  arc A447 (6.6945, 32.1137) -> (5.4258, 29.9297) centre (9.081, 29.267) ccw
  arc A448 (7.0304, 32.0419) -> (6.6945, 32.1137) centre (0, 0) ccw
  arc A449 (7.2944, 29.5299) -> (7.0304, 32.0419) centre (3.6881, 30.4207) ccw
  arc A450 (8.5246, 29.1986) -> (7.2944, 29.5299) centre (0, 0) ccw
  arc A451 (10.0146, 31.2381) -> (8.5246, 29.1986) centre (12.0904, 28.1575) ccw
  arc A452 (10.3412, 31.1315) -> (10.0146, 31.2381) centre (0, 0) ccw
  arc A453 (10.3412, 28.6057) -> (10.3412, 31.1315) centre (6.8477, 29.8686) ccw
  arc A454 (11.53, 28.1475) -> (10.3412, 28.6057) centre (0, 0) ccw
  arc A455 (13.225, 30.0201) -> (11.53, 28.1475) centre (14.9675, 26.7394) ccw
  arc A456 (13.5387, 29.88) -> (13.225, 30.0201) centre (0, 0) ccw
  arc A457 (13.2746, 27.368) -> (13.5387, 29.88) centre (9.9323, 28.9892) ccw
  arc A458 (14.409, 26.7881) -> (13.2746, 27.368) centre (0, 0) ccw
  arc A459 (16.2905, 28.4733) -> (14.409, 26.7881) centre (17.6805, 25.0284) ccw
  arc A460 (16.5878, 28.3011) -> (16.2905, 28.4733) centre (0, 0) ccw
  arc A461 (16.0627, 25.8305) -> (16.5878, 28.3011) centre (12.9081, 27.7921) ccw
  arc A462 (17.1302, 25.1352) -> (16.0627, 25.8305) centre (0, 0) ccw
  arc A463 (19.1776, 26.6145) -> (17.1302, 25.1352) centre (20.1998, 23.0432) ccw
  arc A464 (19.4552, 26.4122) -> (19.1776, 26.6145) centre (0, 0) ccw
  arc A465 (18.6747, 24.01) -> (19.4552, 26.4122) centre (15.7425, 26.2906) ccw
  arc A466 (19.6637, 23.2069) -> (18.6747, 24.01) centre (0, 0) ccw
  arc A467 (21.8545, 24.4641) -> (19.6637, 23.2069) centre (22.4979, 20.8055) ccw
  arc A468 (22.1094, 24.2339) -> (21.8545, 24.4641) centre (0, 0) ccw
  arc A469 (21.0821, 21.9264) -> (22.1094, 24.2339) centre (18.4044, 24.5011) ccw
  arc A470 (21.9818, 21.0244) -> (21.0821, 21.9264) centre (0, 0) ccw
  arc A471 (24.2919, 22.0457) -> (21.9818, 21.0244) centre (24.5494, 18.3399) ccw
  arc A472 (24.5215, 21.7901) -> (24.2919, 22.0457) centre (0, 0) ccw
  arc A473 (23.2586, 19.6026) -> (24.5215, 21.7901) centre (20.8646, 22.4431) ccw
  arc A474 (24.059, 18.6115) -> (23.2586, 19.6026) centre (0, 0) ccw
  arc A475 (26.4633, 19.3857) -> (24.059, 18.6115) centre (26.3319, 15.6733) ccw
  arc A476 (26.6648, 19.1075) -> (26.4633, 19.3857) centre (0, 0) ccw
  arc A477 (25.1802, 17.0641) -> (26.6648, 19.1075) centre (23.0962, 20.1392) ccw
  arc A478 (25.8727, 15.9947) -> (25.1802, 17.0641) centre (0, 0) ccw
  arc A479 (28.3446, 16.5133) -> (25.8727, 15.9947) centre (27.826, 12.835) ccw
  arc A480 (28.516, 16.2156) -> (28.3446, 16.5133) centre (0, 0) ccw
  arc A481 (26.8259, 14.3386) -> (28.516, 16.2156) centre (25.0748, 17.6146) ccw
  arc A482 (27.4028, 13.2026) -> (26.8259, 14.3386) centre (0, 0) ccw
  arc A483 (29.9155, 13.46) -> (27.4028, 13.2026) centre (29.0152, 9.8561) ccw
  arc A484 (30.0548, 13.146) -> (29.9155, 13.46) centre (0, 0) ccw
  arc A485 (28.1778, 11.4559) -> (30.0548, 13.146) centre (26.7787, 14.8971) ccw
  arc A486 (28.6328, 10.2659) -> (28.1778, 11.4559) centre (0, 0) ccw
  arc A487 (31.1586, 10.2593) -> (28.6328, 10.2659) centre (29.8865, 6.7692) ccw
  arc A488 (31.2643, 9.9324) -> (31.1586, 10.2593) centre (0, 0) ccw
  arc A489 (29.2209, 8.4478) -> (31.2643, 9.9324) centre (28.1892, 12.0164) ccw
  arc A490 (29.549, 7.2167) -> (29.2209, 8.4478) centre (0, 0) ccw
  arc A491 (32.0603, 6.9461) -> (29.549, 7.2167) centre (30.4303, 3.6081) ccw
  arc A492 (32.1312, 6.61) -> (32.0603, 6.9461) centre (0, 0) ccw
  arc A493 (29.9438, 5.3471) -> (32.1312, 6.61) centre (29.2908, 9.004) ccw
  arc A494 (30.1415, 4.0885) -> (29.9438, 5.3471) centre (0, 0) ccw
  arc A495 (32.6107, 3.5569) -> (30.1415, 4.0885) centre (30.6408, 0.4075) ccw
  arc A496 (32.6462, 3.2152) -> (32.6107, 3.5569) centre (0, 0) ccw
  arc A497 (30.3387, 2.1878) -> (32.6462, 3.2152) centre (30.0715, 5.8929) ccw
  arc A498 (30.4037, 0.9155) -> (30.3387, 2.1878) centre (0, 0) ccw
  arc A499 (32.8038, 0.1286) -> (30.4037, 0.9155) centre (30.5155, -2.7976) ccw
  arc A500 (32.8034, -0.2149) -> (32.8038, 0.1286) centre (0, 0) ccw
  arc A501 (30.4012, -0.9954) -> (32.8034, -0.2149) centre (30.5228, 2.7173) ccw
  arc A502 (30.3329, -2.2676) -> (30.4012, -0.9954) centre (0, 0) ccw
  arc A503 (32.6376, -3.301) -> (30.3329, -2.2676) centre (30.0559, -5.972) ccw
  arc A504 (32.6012, -3.6426) -> (32.6376, -3.301) centre (0, 0) ccw
  arc A505 (30.1306, -4.1677) -> (32.6012, -3.6426) centre (30.6396, -0.4881) ccw
  arc A506 (29.9297, -5.4258) -> (30.1306, -4.1677) centre (0, 0) ccw
  arc A507 (32.1137, -6.6945) -> (29.9297, -5.4258) centre (29.267, -9.081) ccw
  arc A508 (32.0419, -7.0304) -> (32.1137, -6.6945) centre (0, 0) ccw
  arc A509 (29.5299, -7.2944) -> (32.0419, -7.0304) centre (30.4207, -3.6881) ccw
  arc A510 (29.1986, -8.5246) -> (29.5299, -7.2944) centre (0, 0) ccw
  arc A511 (31.2381, -10.0146) -> (29.1986, -8.5246) centre (28.1575, -12.0904) ccw
  arc A512 (31.1315, -10.3412) -> (31.2381, -10.0146) centre (0, 0) ccw
  arc A513 (28.6057, -10.3412) -> (31.1315, -10.3412) centre (29.8686, -6.8477) ccw
  arc A514 (-19.6657, 20.5138) -> (-25.5542, 12.4313) centre (-7.1656, 5.2205) ccw
  arc A515 (-25.5542, 12.4313) -> (-28.4112, 0.5997) centre (0, 0) ccw
  arc A516 (-28.4112, 0.5997) -> (-26.8598, -9.2793) centre (-8.7583, -1.3754) ccw
  arc A517 (-26.8598, -9.2793) -> (-20.5138, -19.6657) centre (0, 0) ccw
  arc A518 (-20.5138, -19.6657) -> (-12.4313, -25.5542) centre (-5.2205, -7.1656) ccw
  arc A519 (-12.4313, -25.5542) -> (-0.5997, -28.4112) centre (0, 0) ccw
  arc A520 (-0.5997, -28.4112) -> (9.2793, -26.8598) centre (1.3754, -8.7583) ccw
  arc A521 (9.2793, -26.8598) -> (19.6657, -20.5138) centre (0, 0) ccw
  arc A522 (19.6657, -20.5138) -> (25.5542, -12.4313) centre (7.1656, -5.2205) ccw
  arc A523 (25.5542, -12.4313) -> (28.4112, -0.5997) centre (0, 0) ccw
  arc A524 (28.4112, -0.5997) -> (26.8598, 9.2793) centre (8.7583, 1.3754) ccw
  arc A525 (26.8598, 9.2793) -> (20.5138, 19.6657) centre (0, 0) ccw
  arc A526 (20.5138, 19.6657) -> (12.4313, 25.5542) centre (5.2205, 7.1656) ccw
  arc A527 (12.4313, 25.5542) -> (0.5997, 28.4112) centre (0, 0) ccw
  arc A528 (0.5997, 28.4112) -> (-9.2793, 26.8598) centre (-1.3754, 8.7583) ccw
  arc A529 (-9.2793, 26.8598) -> (-19.6657, 20.5138) centre (0, 0) ccw
  arc A530 (-0.0111, -25.713) -> (7.892, -24.4719) centre (3.6693, -23.366) ccw
  arc A531 (7.892, -24.4719) -> (-0.0111, -25.713) centre (3.9404, -25.0925) ccw
  arc A532 (25.713, -0.0111) -> (24.4719, 7.892) centre (23.366, 3.6693) ccw
  arc A533 (24.4719, 7.892) -> (25.713, -0.0111) centre (25.0925, 3.9404) ccw
  arc A534 (-25.713, 0.0111) -> (-24.4719, -7.892) centre (-23.366, -3.6693) ccw
  arc A535 (-24.4719, -7.892) -> (-25.713, 0.0111) centre (-25.0925, -3.9404) ccw
  circle A536 centre (-1.9702, 12.5462) radius 3.75
  circle A537 centre (-1.9702, 12.5462) radius 2.2225
  circle A538 centre (-12.5462, -1.9702) radius 3.75
  circle A539 centre (-12.5462, -1.9702) radius 2.2225
  circle A540 centre (1.9702, -12.5462) radius 3.75
  circle A541 centre (1.9702, -12.5462) radius 2.2225
  circle A542 centre (12.5462, 1.9702) radius 3.75
  circle A543 centre (12.5462, 1.9702) radius 2.2225
  arc A544 (5.316, 3.4059) -> (1.6126, 6.1041) centre (2.1152, 2.9033) ccw
  line L0 (1.6126, 6.1041) -> (-3.4059, 5.316)
  arc A545 (-3.4059, 5.316) -> (-6.1041, 1.6126) centre (-2.9033, 2.1152) ccw
  line L1 (-6.1041, 1.6126) -> (-5.316, -3.4059)
  arc A546 (-5.316, -3.4059) -> (-1.6126, -6.1041) centre (-2.1152, -2.9033) ccw
  line L2 (-1.6126, -6.1041) -> (3.4059, -5.316)
  arc A547 (3.4059, -5.316) -> (6.1041, -1.6126) centre (2.9033, -2.1152) ccw
  line L3 (6.1041, -1.6126) -> (5.316, 3.4059)
  arc A548 (3.0018, -2.7425) -> (3.5306, -2.0167) centre (2.9033, -2.1152) ccw
  line L4 (3.0018, -2.7425) -> (-2.0167, -3.5306)
  arc A549 (-2.7425, -3.0018) -> (-2.0167, -3.5306) centre (-2.1152, -2.9033) ccw
  line L5 (-2.7425, -3.0018) -> (-3.5306, 2.0167)
  arc A550 (-3.0018, 2.7425) -> (-3.5306, 2.0167) centre (-2.9033, 2.1152) ccw
  line L6 (-3.0018, 2.7425) -> (2.0167, 3.5306)
  arc A551 (2.7425, 3.0018) -> (2.0167, 3.5306) centre (2.1152, 2.9033) ccw
  line L7 (2.7425, 3.0018) -> (3.5306, -2.0167)
  constraints: 1072 point on circle, 552 centre point, 16 end point
extrude "Extrusion1" add sketch "Sketch1" against normal blind 12.7 contours A239 A238 A237 A236 A235 A234 A233 A232 A231 A230 A229 A228 A227 A226 A225 A224 A223 A222 A221 A220 A219 A218 A217 A216 A215 A214 A213 A212 A211 A210 A209 A208 A207 A206 A205 A204 A203 A202 A201 A200 A199 A198 A197 A196 A195 A194 A193 A192 A191 A190 A189 A188 A187 A186 A185 A184 A183 A182 A181 A180 A179 A178 A177 A176 A175 A174 A173 A172 A171 A170 A169 A168 A167 A166 A165 A164 A163 A162 A161 A160 A159 A158 A157 A156 A155 A154 A153 A152 A151 A150 A149 A148 A147 A146 A145 A144 A143 A142 A141 A140 A139 A138 A137 A136 A135 A134 A133 A132 A131 A130 A129 A128 A127 A126 A125 A124 A123 A122 A121 A120 A119 A118 A117 A116 A115 A114 A113 A112 A111 A110 A109 A108 A107 A106 A105 A104 A103 A102 A101 A100 A99 A98 A97 A96 A95 A94 A93 A92 A91 A90 A89 A88 A87 A86 A85 A84 A83 A82 A81 A80 A79 A78 A77 A76 A75 A74 A73 A72 A71 A70 A69 A68 A67 A66 A65 A64 A63 A62 A61 A60 A59 A58 A57 A56 A55 A54 A53 A52 A51 A50 A49 A48 A47 A46 A45 A44 A43 A42 A41 A40 A39 A38 A37 A36 A35 A34 A33 A32 A31 A30 A29 A28 A27 A26 A25 A24 A23 A22 A21 A20 A19 A18 A17 A16 A15 A14 A13 A12 A11 A10 A9 A8 A7 A6 A5 A4 A3 A2 A1 A0
ref_plane "Work Plane1" through (0, 0, -5.2578) normal (0, 0, 1) x (1, 0, 0)
ref_plane "Work Plane2" through (0, 0, -7.4422) normal (0, 0, -1) x (-1, 0, 0)
extrude "Extrusion2" add sketch "Sketch1" against normal up to surface (2.1844 mm away) from surface at -5.2578 contours A241 A242 A243 A244 A245 A246 A247 A248 A249 A250 A251 A252 A253 A254 A255 A240
extrude "Extrusion3" add sketch "Sketch1" against normal up to surface (12.7 mm away) contours A257 A256 | A259 A258 | A261 A260 | A263 A262 | A265 A264 | A266 | A267 | A268 | A269 | A270 | A271 | A272 | A273 | A531 A530 | A533 A532 | A535 A534
extrude "Extrusion4" cut sketch "Sketch1" against normal up to surface (12.7 mm away) contours A266 | A267 | A268 | A269 | A270 | A271 | A272 | A273
ref_plane "Work Plane3" through (0, 0, -4.7752) normal (0, 0, 1) x (0.9720622, -0.2347236, 0)
ref_plane "Work Plane4" through (0, 0, -7.9248) normal (0, 0, -1) x (-0.8533264, -0.5213771, 0)
extrude "Extrusion5" add sketch "Sketch1" along normal up to surface (3.1496 mm away) from surface at -7.9248 contours A536 | A537 | A538 | A539 | A540 | A541 | A542 | A543
extrude "Extrusion6" cut sketch "Sketch1" against normal up to surface (3.1496 mm away) from surface at -4.7752 contours A537 | A539 | A541 | A543
sketch "Sketch2" plane through (0, 0, -5.2578) normal (0, 0, 1) x (0.9720622, -0.2347236, 0)
  line L0 (0.1347, 6.312) -> (-4.5586, 4.368) projected
  arc A0 (4.368, 4.5586) -> (0.1347, 6.312) centre (1.3746, 3.3187) ccw projected
  line L1 (6.312, -0.1347) -> (4.368, 4.5586) projected
  arc A1 (4.5586, -4.368) -> (6.312, -0.1347) centre (3.3187, -1.3746) ccw projected
  line L2 (-0.1347, -6.312) -> (4.5586, -4.368) projected
  arc A2 (-4.368, -4.5586) -> (-0.1347, -6.312) centre (-1.3746, -3.3187) ccw projected
  line L3 (-6.312, 0.1347) -> (-4.368, -4.5586) projected
  arc A3 (-4.5586, 4.368) -> (-6.312, 0.1347) centre (-3.3187, 1.3746) ccw projected
extrude "Extrusion7" add sketch "Sketch2" along normal blind 3.78 and the other way blind 5.98
extrude "Extrusion8" cut sketch "Sketch1" against normal up to surface (11.2378 mm away) contours L4 A549 L5 A550 L6 A551 L7 A548
sketch "Sketch3" plane through (0, 0, -1.4778) normal (0, 0, 1) x (0.9720622, -0.2347236, 0)
  line L0 (-3.5617, 1.9613) -> (1.1316, 3.9053) projected
  circle A0 centre (0, 0) radius 3.175
  constraints: 1 centre point, 1 coincident, 1 tangent
surface extrude "ExtrusionSrf1" sketch "Sketch3" against normal up to surface (9.76 mm away) shown no curves A0
body "Solid1"
body "Srf1"
